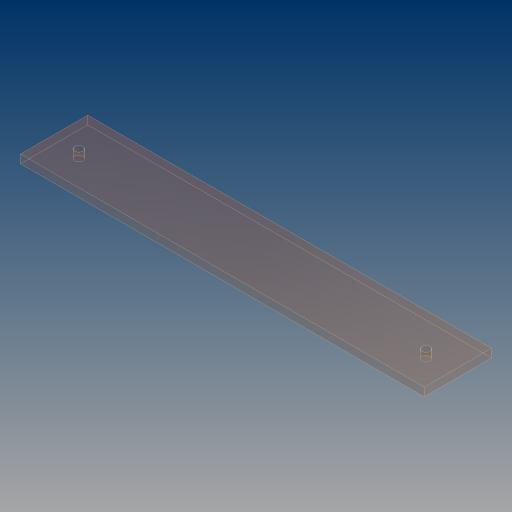
# Autodesk Inventor part: 6holepolycarb
Saved by Autodesk Inventor 2023 (Build 270158000, 158)
## iProperties
Created: 2023-07-17
Part Number: 6holepolycarb
Material: Generic
Document SubType Name: Modeling
Designer: eddie
Density: 1 g/cm^3
Appearance: Polycarbonate - Smoked
Author: eddie
Autodesk Inventor part; units mm, degrees
ref_plane "YZ Plane" through (0, 0, 0) normal (1, 0, 0) x (0, 1, 0)
ref_plane "XZ Plane" through (0, 0, 0) normal (0, 1, 0) x (-1, 0, 0)
ref_plane "XY Plane" through (0, 0, 0) normal (0, 0, 1) x (1, 0, 0)
sketch "Sketch1" plane through (0, 0, 0) normal (0, 1, 0) x (-1, 0, 0)
  line L0 (0, 0) -> (76.2, 0)
  line L1 (76.2, 0) -> (76.2, -12.7)
  line L2 (76.2, -12.7) -> (0, -12.7)
  line L3 (0, -12.7) -> (0, 0)
  dimension "d0" = 76.2
  dimension "d1" = 12.7
  constraints: 8 end point, 2 parallel, 1 horizontal, 1 perpendicular
  measures "d0" distance of L1.end L2.end
  measures "d1" distance of L0.end L1.end
sketch "Sketch2" plane through (0, 0, 0) normal (0, 1, 0) x (-1, 0, 0)
  circle A0 centre (71.5517, -6.3478) radius 0.7937
  line L0 (70.7579, -6.3478) -> (7.2579, -6.3478)
  circle A1 centre (6.0742, -6.4004) radius 0.7937
  point P0 (0, 0)
  point P1 (72.2309, -10.2346)
  point P2 (6.6877, -6.9041)
  dimension "d2" = 1.5875
  dimension "d6" = 1.5875
  dimension "d3" = 63.5
  constraints: 2 end point, 1 horizontal, 1 horizontal alignment, 5 other
  measures "d3" distance of L0.start L0.end
extrude "Extrusion1" add sketch "Sketch1" along normal blind 1.5875
extrude "Extrusion2" cut sketch "Sketch2" along normal blind 1.5875
body "Solid1"
